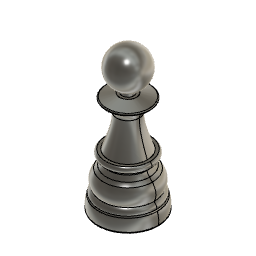
Pawn v1 (Autodesk Fusion 360 design; units mm, degrees)
Autodesk Fusion 360 part; units mm, degrees
sketch "Sketch1" plane through (0, 0, 0) normal (0, 1, 0) x (1, 0, 0)
  line L0 (0, 0) -> (0, -22)
  line L1 (0.80644, -14.746362) -> (0.80644, -14.207459)
  line L2 (0.80644, -14.207459) -> (1.172124, -14.207459)
  line L3 (1.172124, -14.207459) -> (2.92776, -13.754975)
  line L4 (3.039039, -13.61138) -> (3.039039, -13.616845)
  line L5 (2.915248, -13.45168) -> (2.31358, -13.27577)
  line L6 (2.676309, -7.448927) -> (3.072214, -7.448927)
  line L7 (3.072214, -6.600535) -> (2.774728, -6.458939)
  line L8 (3.970889, -2.14419) -> (4.060049, -1.956869)
  line L9 (0, 0) -> (3.747856, 0)
  arc A0 (2.963996, -13.745636) -> (3.039039, -13.648801) centre (2.939039, -13.648801) ccw
  arc A1 (2.92776, -13.754975) -> (3.039039, -13.61138) centre (2.89075, -13.61138) ccw
  arc A2 (3.039039, -13.616845) -> (2.915248, -13.45168) centre (2.866958, -13.616845) ccw
  spline S0 degree 5 poles (2.31358, -13.27577) (2.267684, -13.221904) (2.177784, -13.114116) (2.048614, -12.952268) (1.888533, -12.736111) (1.71858, -12.465028) (1.621933, -12.247003) (1.582671, -12.082505) (1.573625, -11.972336) (1.573388, -11.917125) knots 0 0 0 0 0 0 0.2 0.4 0.6 0.8 1 1 1 1 1 1
  line L10 (1.57401, -12.061997) -> (1.572766, -11.772252)
  spline S1 degree 5 poles (1.642131, -11.502154) (1.642131, -11.502154) (1.642132, -11.502153) (1.642132, -11.502152) (1.642133, -11.50215) (1.642134, -11.502148) (1.642134, -11.502146) (1.642135, -11.502144) (1.642135, -11.502144) (1.642135, -11.502143) knots 0 0 0 0 0 0 0.2 0.4 0.6 0.8 1 1 1 1 1 1
  line L11 (1.642131, -11.502156) -> (1.642132, -11.502153)
  line L12 (1.642135, -11.502144) -> (1.642135, -11.502142)
  spline S2 degree 5 poles (2.676309, -7.448927) (2.607281, -7.62314) (2.47212, -7.972092) (2.278063, -8.497093) (2.037898, -9.200461) (1.783798, -10.088027) (1.640646, -10.808976) (1.584092, -11.358896) (1.572586, -11.730256) (1.573388, -11.917125) knots 0 0 0 0 0 0 0.2 0.4 0.6 0.8 1 1 1 1 1 1
  spline S3 degree 5 poles (3.072214, -7.448927) (3.114999, -7.422048) (3.190986, -7.36671) (3.276237, -7.278963) (3.337981, -7.153404) (3.340634, -6.984163) (3.281295, -6.838634) (3.194929, -6.722582) (3.116583, -6.641789) (3.072214, -6.600535) knots 0 0 0 0 0 0 0.2 0.4 0.6 0.8 1 1 1 1 1 1
  line L13 (3.176557, -6.697551) -> (2.96787, -6.503519)
  spline S4 degree 5 poles (2.987854, -5.527156) (3.106073, -5.426747) (3.320425, -5.225109) (3.57575, -4.920192) (3.797758, -4.50905) (3.913566, -3.98761) (3.882264, -3.563199) (3.778558, -3.239474) (3.670038, -3.020923) (3.605925, -2.910963) knots 0 0 0 0 0 0 0.2 0.4 0.6 0.8 1 1 1 1 1 1
  line L14 (3.767064, -3.187331) -> (3.444785, -2.634594)
  spline S5 degree 5 poles (2.629909, -6.129464) (2.63674, -6.107255) (2.652483, -6.061853) (2.682347, -5.990796) (2.733644, -5.891204) (2.811503, -5.764335) (2.896711, -5.641857) (2.983546, -5.529675) (3.068493, -5.430872) (3.152025, -5.343275) (3.237153, -5.261586) (3.309772, -5.195921) (3.368434, -5.144061) (3.409649, -5.10799) (3.430782, -5.089581) knots 0 0 0 0 0 0 0.1 0.2 0.3 0.4 0.5 0.6 0.7 0.8 0.9 1 1 1 1 1 1
  line L15 (3.286705, -5.215088) -> (3.574859, -4.964074)
  arc A3 (2.629909, -6.129464) -> (2.774728, -6.458939) centre (2.89304, -6.210372) ccw
  arc A4 (4.232341, -0.37641) -> (3.747856, 0) centre (3.747856, -0.5) ccw
  spline S6 degree 5 poles (4.060049, -1.956869) (4.086226, -1.899123) (4.133739, -1.780937) (4.190481, -1.595576) (4.238793, -1.336467) (4.26289, -1.016066) (4.262223, -0.728254) (4.248376, -0.500757) (4.231137, -0.352534) (4.216654, -0.284876) (4.205637, -0.271612) (4.197785, -0.274693) (4.191049, -0.269332) (4.185945, -0.260148) (4.18324, -0.254152) knots 0 0 0 0 0 0 0.1 0.2 0.3 0.4 0.5 0.6 0.7 0.8 0.9 1 1 1 1 1 1
  line L16 (4.257133, -0.417941) -> (4.109348, -0.090363)
  spline S7 degree 5 poles (3.605925, -2.910963) (3.646901, -2.881589) (3.723128, -2.822559) (3.820304, -2.73317) (3.918654, -2.612451) (3.99546, -2.459284) (4.017355, -2.334806) (4.006167, -2.24009) (3.984944, -2.17627) (3.970889, -2.14419) knots 0 0 0 0 0 0 0.2 0.4 0.6 0.8 1 1 1 1 1 1
  spline S8 degree 5 poles (-3.605925, -2.910963) (-3.646901, -2.881589) (-3.723128, -2.822559) (-3.820304, -2.73317) (-3.918654, -2.612451) (-3.99546, -2.459284) (-4.017355, -2.334806) (-4.006167, -2.24009) (-3.984944, -2.17627) (-3.970889, -2.14419) knots 0 0 0 0 0 0 0.2 0.4 0.6 0.8 1 1 1 1 1 1
  line L17 (3.491287, -2.993141) -> (3.720563, -2.828784)
  line L18 (4.006509, -2.225489) -> (3.935268, -2.062892)
  line L19 (-3.491287, -2.993141) -> (-3.720563, -2.828784)
  line L20 (-4.006509, -2.225489) -> (-3.935268, -2.062892)
  spline S9 degree 5 poles (-4.060049, -1.956869) (-4.086226, -1.899123) (-4.133739, -1.780937) (-4.190481, -1.595576) (-4.238793, -1.336467) (-4.26289, -1.016066) (-4.262223, -0.728254) (-4.248376, -0.500757) (-4.231137, -0.352534) (-4.216654, -0.284876) (-4.205637, -0.271612) (-4.197785, -0.274693) (-4.191049, -0.269332) (-4.185945, -0.260148) (-4.18324, -0.254152) knots 0 0 0 0 0 0 0.1 0.2 0.3 0.4 0.5 0.6 0.7 0.8 0.9 1 1 1 1 1 1
  line L21 (3.974561, -2.145451) -> (4.145537, -1.768288)
  line L22 (-3.974561, -2.145451) -> (-4.145537, -1.768288)
  line L23 (-4.257133, -0.417941) -> (-4.109348, -0.090363)
  line L24 (0, 0) -> (-3.747856, 0)
  arc A5 (-3.747856, 0) -> (-4.232341, -0.37641) centre (-3.747856, -0.5) ccw
  spline S10 degree 5 poles (-1.642131, -11.502154) (-1.642131, -11.502154) (-1.642132, -11.502153) (-1.642132, -11.502152) (-1.642133, -11.50215) (-1.642134, -11.502148) (-1.642134, -11.502146) (-1.642135, -11.502144) (-1.642135, -11.502144) (-1.642135, -11.502143) knots 0 0 0 0 0 0 0.2 0.4 0.6 0.8 1 1 1 1 1 1
  line L25 (-1.642131, -11.502156) -> (-1.642132, -11.502153)
  line L26 (-1.642135, -11.502144) -> (-1.642135, -11.502142)
  line L27 (-3.970889, -2.14419) -> (-4.060049, -1.956869)
  spline S11 degree 5 poles (-2.676309, -7.448927) (-2.607281, -7.62314) (-2.47212, -7.972092) (-2.278063, -8.497093) (-2.037898, -9.200461) (-1.783798, -10.088027) (-1.640646, -10.808976) (-1.584092, -11.358896) (-1.572586, -11.730256) (-1.573388, -11.917125) knots 0 0 0 0 0 0 0.2 0.4 0.6 0.8 1 1 1 1 1 1
  line L28 (2.856024, -6.995365) -> (2.496595, -7.902489)
  line L29 (1.571322, -11.435659) -> (1.575454, -12.398591)
  line L30 (-2.856024, -6.995365) -> (-2.496595, -7.902489)
  line L31 (-1.571322, -11.435659) -> (-1.575454, -12.398591)
  line L32 (-2.676309, -7.448927) -> (-3.072214, -7.448927)
  spline S12 degree 5 poles (-2.31358, -13.27577) (-2.267684, -13.221904) (-2.177784, -13.114116) (-2.048614, -12.952268) (-1.888533, -12.736111) (-1.71858, -12.465028) (-1.621933, -12.247003) (-1.582671, -12.082505) (-1.573625, -11.972336) (-1.573388, -11.917125) knots 0 0 0 0 0 0 0.2 0.4 0.6 0.8 1 1 1 1 1 1
  line L33 (2.43988, -13.424001) -> (2.18728, -13.127539)
  line L34 (-2.43988, -13.424001) -> (-2.18728, -13.127539)
  line L35 (-1.57401, -12.061997) -> (-1.572766, -11.772252)
  arc A6 (-3.039039, -13.61138) -> (-2.92776, -13.754975) centre (-2.89075, -13.61138) ccw
  arc A7 (-3.039039, -13.648801) -> (-2.963996, -13.745636) centre (-2.939039, -13.648801) ccw
  line L36 (-3.039039, -13.61138) -> (-3.039039, -13.616845)
  line L37 (-1.172124, -14.207459) -> (-2.92776, -13.754975)
  line L38 (-0.80644, -14.207459) -> (-1.172124, -14.207459)
  line L39 (-0.80644, -14.746362) -> (-0.80644, -14.207459)
  spline S13 degree 5 poles (-2.987854, -5.527156) (-3.106073, -5.426747) (-3.320425, -5.225109) (-3.57575, -4.920192) (-3.797758, -4.50905) (-3.913566, -3.98761) (-3.882264, -3.563199) (-3.778558, -3.239474) (-3.670038, -3.020923) (-3.605925, -2.910963) knots 0 0 0 0 0 0 0.2 0.4 0.6 0.8 1 1 1 1 1 1
  line L40 (2.679853, -5.788756) -> (3.295855, -5.265557)
  line L41 (-2.679853, -5.788756) -> (-3.295855, -5.265557)
  line L42 (-3.767064, -3.187331) -> (-3.444785, -2.634594)
  arc A8 (-2.774728, -6.458939) -> (-2.629909, -6.129464) centre (-2.89304, -6.210372) ccw
  spline S14 degree 5 poles (-3.072214, -7.448927) (-3.114999, -7.422048) (-3.190986, -7.36671) (-3.276237, -7.278963) (-3.337981, -7.153404) (-3.340634, -6.984163) (-3.281295, -6.838634) (-3.194929, -6.722582) (-3.116583, -6.641789) (-3.072214, -6.600535) knots 0 0 0 0 0 0 0.2 0.4 0.6 0.8 1 1 1 1 1 1
  line L43 (2.977668, -7.508323) -> (3.166759, -7.389531)
  line L44 (-2.977668, -7.508323) -> (-3.166759, -7.389531)
  line L45 (-3.176557, -6.697551) -> (-2.96787, -6.503519)
  spline S15 degree 5 poles (-2.629909, -6.129464) (-2.63674, -6.107255) (-2.652483, -6.061853) (-2.682347, -5.990796) (-2.733644, -5.891204) (-2.811503, -5.764335) (-2.896711, -5.641857) (-2.983546, -5.529675) (-3.068493, -5.430872) (-3.152025, -5.343275) (-3.237153, -5.261586) (-3.309772, -5.195921) (-3.368434, -5.144061) (-3.409649, -5.10799) (-3.430782, -5.089581) knots 0 0 0 0 0 0 0.1 0.2 0.3 0.4 0.5 0.6 0.7 0.8 0.9 1 1 1 1 1 1
  line L46 (2.588149, -6.265248) -> (2.67167, -5.99368)
  line L47 (-2.588149, -6.265248) -> (-2.67167, -5.99368)
  line L48 (-3.286705, -5.215088) -> (-3.574859, -4.964074)
  line L49 (-3.072214, -6.600535) -> (-2.774728, -6.458939)
  line L50 (-2.915248, -13.45168) -> (-2.31358, -13.27577)
  arc A9 (-2.915248, -13.45168) -> (-3.039039, -13.616845) centre (-2.866958, -13.616845) ccw
  arc A10 (-0.80644, -14.746362) -> (0.80644, -14.746362) centre (0, -17.250034) ccw
  dimension "d1" = 0.1
  dimension "d2" = 0.148288
  dimension "d3" = 0.17208
  dimension "d4" = 0.275288
  dimension "d5" = 0.5
  constraint vertical L0
  constraint parallel L0 L1
  constraint perpendicular L1 L2
  constraint perpendicular L2 L4
  constraint perpendicular L1 L6
  constraint perpendicular L0 L9
  constraint tangent L3 A0
  constraint tangent L4 A0
  constraint tangent L3 A1
  constraint tangent L4 A1
  constraint tangent L5 A2
  constraint tangent L4 A2
  constraint tangent S5 A3
  constraint tangent L7 A3
  constraint tangent L9 A4
  constraint symmetric L9.start L0 L24.start
  constraint symmetric L0 A0 A7
  constraint symmetric L0 A1 A6
  constraint symmetric L0 A2 A9
  constraint symmetric L0 A3 A8
  constraint symmetric L0 A4 A5
  measures "d1" radius of A0
  measures "d2" radius of A1
  measures "d3" radius of A2
  measures "d4" radius of A3
  measures "d5" radius of A4
sketch "Sketch2" plane through (0, 0, 0) normal (0, 1, 0) x (1, 0, 0)
revolve "Revolve1" add sketch "Sketch1" angle 360 about axis through (0, 0, 0) along (0, 0, 1) contours L0 L1 L2 L3 L4 L5 L6 L7 L8 L9 A1 A2 S0 L10 S2 S3 S4 S5 L15 A3 A4 S6 L16 S7 L29 A10 picked at (2.197926, -2.812706)
